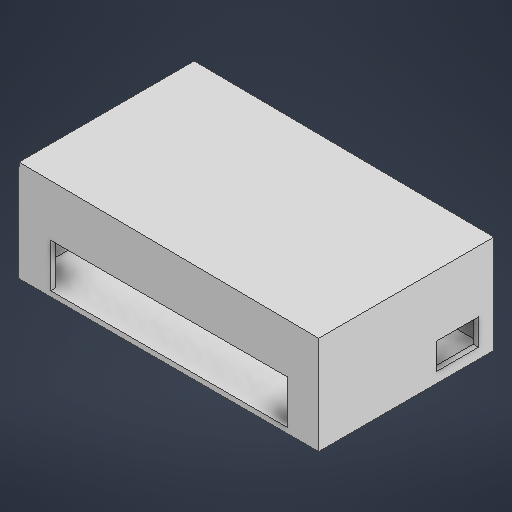
# Autodesk Inventor part: Main
Saved by Autodesk Inventor 2027.1 (Build 311270010, 270A)
## iProperties
Created: 2026-09-11
Part Number: Main
Material: Generic
Document SubType Name: Modeling
Designer: thaua
Density: 1 g/cm^3
Appearance: Default
Author: thaua
Autodesk Inventor part; units mm, degrees
ref_plane "YZ Plane" through (0, 0, 0) normal (1, 0, 0) x (0, 1, 0)
ref_plane "XZ Plane" through (0, 0, 0) normal (0, 1, 0) x (-1, 0, 0)
ref_plane "XY Plane" through (0, 0, 0) normal (0, 0, 1) x (1, 0, 0)
sketch "Sketch1" plane through (0, 0, 0) normal (0, 0, 1) x (1, 0, 0)
  line L0 (-16.8678, 0) -> (148.1322, 0)
  line L1 (-16.8678, 0) -> (-16.8678, 50)
  line L2 (-16.8678, 50) -> (148.1322, 50)
  line L3 (148.1322, 50) -> (148.1322, 0)
  line L4 (-16.8678, 0) -> (-16.8678, -3)
  line L5 (-16.8678, -3) -> (151.1322, -3)
  line L6 (151.1322, -3) -> (151.1322, 50)
  line L7 (151.1322, 50) -> (151.1322, 53)
  line L8 (151.1322, 53) -> (-19.8606, 54.5715)
  line L9 (-19.8606, 54.5715) -> (-20.3897, -3)
  arc A0 (-20.3897, -3) -> (-16.8678, -3) centre (-18.6288, 188.6018) ccw
  point P0 (0, 0)
  dimension "d0" = 165
  dimension "d2" = 50
  dimension "d3" = 165
  dimension "d4" = 3
  dimension "d5" = 168
  dimension "d6" = 53
  dimension "d7" = 3
  dimension "d8" = 171
  constraints: 20 end point, 4 perpendicular, 3 point on line, 2 point on circle, 2 vertical, 1 centre point, 1 horizontal
  measures "d0" distance of L0.start L0.end
  measures "d2" distance of L0.start L1.end
  measures "d3" distance of L1.end L2.end
  measures "d4" distance of L0.start L4.end
  measures "d5" distance of L4.end L5.end
  measures "d6" distance of L5.end L6.end
  measures "d7" distance of L6.end L7.end
  measures "d8" distance of L7.end L8.end
extrude "Extrusion1" add sketch "Sketch1" along normal blind 100
sketch "Sketch2" plane through (0, 0, 100) normal (0, 0, 1) x (1, 0, 0)
  line L0 (148.1322, 0) -> (-16.8678, 0) projected
  line L1 (-16.8678, 0) -> (-1.8678, 0)
  line L2 (-1.8678, 0) -> (-1.8678, 3.4426)
  line L3 (-1.8678, 0) -> (-1.8678, 25)
  line L4 (-1.8678, 25) -> (133.1322, 25)
  line L5 (133.1322, 25) -> (133.1322, 0)
  line L6 (-16.8678, 0) -> (-16.8678, 50)
  line L7 (-16.8678, 50) -> (148.1322, 50)
  line L8 (148.1322, 50) -> (148.1322, 0)
  line L9 (148.1322, 0) -> (133.1322, 0)
  point P0 (0, 0)
  dimension "d11" = 15
  dimension "d12" = 25
  dimension "d13" = 135
  dimension "d14" = 50
  dimension "d15" = 165
  dimension "d16" = 50
  constraints: 18 end point, 4 perpendicular, 2 point on line, 1 vertical
  measures "d11" distance of L0.end L1.end
  measures "d12" distance of L1.end L3.end
  measures "d13" distance of L3.end L4.end
  measures "d14" distance of L0.end L6.end
  measures "d15" distance of L6.end L7.end
  measures "d16" distance of L7.end L0.start
extrude "Extrusion2" add sketch "Sketch2" against normal blind 3 contours L0 L5 L4 L3 L2 L6 L7 L8
sketch "Sketch3" plane through (0, 0, 0) normal (0, 0, -1) x (-1, 0, 0)
  line L0 (-148.1322, 0) -> (16.8678, 0) projected
  line L1 (-148.1322, 0) -> (16.8678, 0)
  line L2 (16.8678, 0) -> (16.8678, 50)
  line L3 (16.8678, 50) -> (-148.1322, 50)
  line L4 (-148.1322, 50) -> (-148.1322, 0)
  point P0 (0, 0)
  dimension "d19" = 165
  dimension "d20" = 50
  dimension "d21" = 165
  constraints: 8 end point, 2 perpendicular, 1 collinear
  measures "d19" distance of L0.start L0.end
  measures "d20" distance of L0.end L2.end
  measures "d21" distance of L2.end L3.end
extrude "Extrusion3" add sketch "Sketch3" against normal blind 3
sketch "Sketch4" plane through (151.1322, -3, 0) normal (1, 0, 0) x (0, 0, -1)
  line L0 (-32.782, 20.9659) -> (-8.782, 20.9659)
  line L1 (-8.782, 20.9659) -> (-8.782, 5.9659)
  line L2 (-8.782, 5.9659) -> (-32.782, 5.9659)
  line L3 (-32.782, 5.9659) -> (-32.782, 20.9659)
  point P0 (0, 3)
  dimension "d24" = 24
  dimension "d25" = 15
  constraints: 8 end point, 2 parallel, 1 horizontal, 1 perpendicular
  measures "d24" distance of L1.end L2.end
  measures "d25" distance of L0.end L1.end
extrude "Extrusion4" cut sketch "Sketch4" against normal blind 3
body "Solid1"
